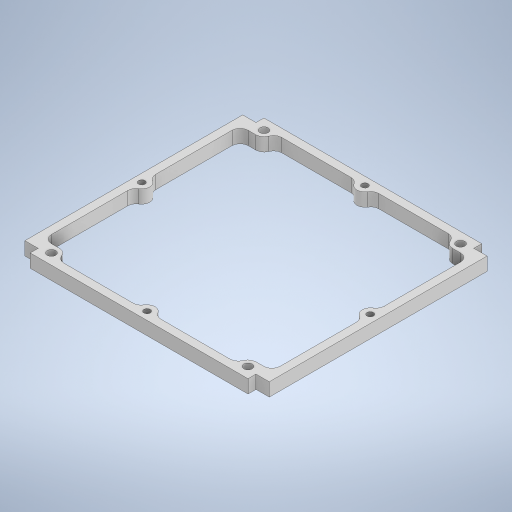
# Autodesk Inventor part: ElectronicsBayUpperMount
Saved by Autodesk Inventor 2023 (Build 270158000, 158)
## iProperties
Created: 2022-08-18
Part Number: ElectronicsBayUpperMount
Material: Generic
Document SubType Name: Modeling
Designer: Aditya Bansal
Density: 1 g/cm^3
Appearance: Default
Author: Aditya Bansal
Autodesk Inventor part; units mm, degrees
ref_plane "YZ Plane" through (0, 0, 0) normal (1, 0, 0) x (0, 1, 0)
ref_plane "XZ Plane" through (0, 0, 0) normal (0, 1, 0) x (-1, 0, 0)
ref_plane "XY Plane" through (0, 0, 0) normal (0, 0, 1) x (1, 0, 0)
sketch "Sketch1" plane through (0, 0, 0) normal (0, 1, 0) x (-1, 0, 0)
  line L0 (0, 0) -> (-92, 0)
  line L1 (-92, 0) -> (-92, -88)
  line L2 (-92, -88) -> (0, -88)
  line L3 (0, -88) -> (0, 0)
  line L4 (0, -88) -> (-5, -88)
  line L5 (-5, -88) -> (-5, -85)
  line L6 (-5, -85) -> (0, -85)
  line L7 (0, -85) -> (0, -88)
  line L8 (0, 0) -> (-5, 0)
  line L9 (-5, 0) -> (-5, -3)
  line L10 (-5, -3) -> (0, -3)
  line L11 (0, -3) -> (0, 0)
  line L12 (-92, 0) -> (-87, 0)
  line L13 (-87, 0) -> (-87, -3)
  line L14 (-87, -3) -> (-92, -3)
  line L15 (-92, -3) -> (-92, 0)
  line L16 (-92, -88) -> (-87, -88)
  line L17 (-87, -88) -> (-87, -85)
  line L18 (-87, -85) -> (-92, -85)
  line L19 (-92, -85) -> (-92, -88)
  circle A0 centre (-9, -84) radius 1.6 construction
  circle A1 centre (-83, -84) radius 1.6 construction
  circle A2 centre (-9, -4) radius 1.6 construction
  circle A3 centre (-83, -4) radius 1.6 construction
  circle A4 centre (-46, -85) radius 1.6 construction
  circle A5 centre (-3, -44) radius 1.6 construction
  circle A6 centre (-89, -44) radius 1.6 construction
  circle A7 centre (-46, -3) radius 1.6 construction
  circle A8 centre (-9, -84) radius 3
  circle A9 centre (-46, -85) radius 3
  circle A10 centre (-83, -84) radius 3
  circle A11 centre (-3, -44) radius 3
  circle A12 centre (-9, -4) radius 3
  circle A13 centre (-83, -4) radius 3
  circle A14 centre (-89, -44) radius 3
  circle A15 centre (-46, -3) radius 3
  line L20 (-11.8284, -3) -> (-43, -3)
  line L21 (-49, -3) -> (-80.1716, -3)
  line L22 (-83, -7) -> (-89, -7)
  line L23 (-89, -7) -> (-89, -41)
  line L24 (-83, -81) -> (-89, -81)
  line L25 (-89, -81) -> (-89, -47)
  line L26 (-80.1716, -85) -> (-49, -85)
  line L27 (-43, -85) -> (-11.8284, -85)
  line L28 (-9, -81) -> (-3, -81)
  line L29 (-9, -7) -> (-3, -7)
  line L30 (-3, -7) -> (-3, -41)
  line L31 (-3, -47) -> (-3, -81)
  point P0 (-92, -44)
  point P1 (-46, 0)
  dimension "d0" = 82
  dimension "d1" = 88
  dimension "d2" = 92
  dimension "d3" = 5
  dimension "d4" = 3.2
  dimension "d5" = 74
  dimension "d6" = 80
  dimension "d7" = 9
  dimension "d8" = 4
  dimension "d9" = 3.2
  dimension "d10" = 46
  dimension "d11" = 44
  dimension "d12" = 3
  dimension "d13" = 3
  dimension "d14" = 3
  dimension "d15" = 3
  dimension "d16" = 6
  dimension "d17" = 3
  dimension "d18" = 3
  dimension "d19" = 3
  dimension "d20" = 3
  constraints: 64 end point, 16 centre point, 16 point on circle, 13 equal radius, 12 parallel, 9 coincident, 8 horizontal, 8 perpendicular, 6 equal length, 6 point on line, 4 collinear, 3 horizontal alignment, 3 vertical alignment, 2 tangent
  measures "d0" distance between parallel lines of L14 L18
  measures "d1" distance between parallel lines of L2 L0
  measures "d2" distance between parallel lines of L3 L1
  measures "d3" distance of L18.start L18.end
  measures "d4" diameter of A0
  measures "d5" distance of A1.centre A0.centre
  measures "d6" distance of A2.centre A0.centre
  measures "d7" distance from line of A0.centre L3
  measures "d8" distance from line of L0 A2.centre
  measures "d9" diameter of A7
  measures "d10" distance from line of L1 A7.centre
  measures "d11" distance from line of L2 A6.centre
  measures "d12" distance from line of L0 A7.centre
  measures "d13" distance from line of L2 A4.centre
  measures "d14" distance from line of L1 A6.centre
  measures "d15" distance from line of L3 A5.centre
  measures "d16" diameter of A12
  measures "d17" distance between parallel lines of L0 L20
  measures "d18" distance between parallel lines of L3 L30
  measures "d19" distance between parallel lines of L27 L2
  measures "d20" distance between parallel lines of L1 L25
extrude "Extrusion1" add sketch "Sketch1" along normal blind 5 contours L9 L10 L3 A11 L30 L29 A12 L20 A15 L0 | A15 L21 A13 L22 L23 A14 L1 L14 L13 L0 | A15 | A11 | L3 L6 L5 L2 A9 L27 A8 L28 L31 A11 | A12 | A13 | A8 | A14 L25 L24 A10 L26 A9 L2 L17 L18 L1 | A14 | A9 | A10
fillet "Fillet1" radius 3 16 edges at (3, 2.5, -7) (11.8284, 2.5, -3) (43, 2.5, -3) (49, 2.5, -3) (80.1716, 2.5, -3) (89, 2.5, -7) (89, 2.5, -41) (89, 2.5, -47) (3, 2.5, -41) (3, 2.5, -47) (3, 2.5, -81) (11.8284, 2.5, -85) (43, 2.5, -85) (49, 2.5, -85) (89, 2.5, -81) (80.1716, 2.5, -85)
sketch "Sketch2" plane through (0, 5, 0) normal (0, 1, 0) x (1, 0, 0)
  arc A0 (87.5, 46.5981) -> (87.5, 41.4019) centre (89, 44) ccw projected
  arc A1 (43.4019, 83.5) -> (48.5981, 83.5) centre (46, 85) ccw projected
  arc A2 (4.5, 41.4019) -> (4.5, 46.5981) centre (3, 44) ccw projected
  arc A3 (48.5981, 4.5) -> (43.4019, 4.5) centre (46, 3) ccw projected
  point P0 (0, 0)
  point P1 (92, 44)
  point P2 (46, 0)
  constraints: 4 coincident
hole "Hole1" at (46, 5, -85) at (3, 5, -44) at (89, 5, -44) at (46, 5, -3) direction (0, -1, 0) diameter 2.459 end through all thread size "M3x0.5" class "6H" standard "ANSI Metric M Profile"
sketch "Sketch3" plane through (0, 5, 0) normal (0, 1, 0) x (1, 0, 0)
  arc A0 (9, 81) -> (11.8284, 83) centre (9, 84) ccw projected
  arc A1 (11.8284, 5) -> (9, 7) centre (9, 4) ccw projected
  arc A2 (80.1716, 83) -> (83, 81) centre (83, 84) ccw projected
  arc A3 (83, 7) -> (80.1716, 5) centre (83, 4) ccw projected
  point P0 (0, 0)
  point P1 (84, 6)
  constraints: 4 coincident, 1 other
hole "Hole2" at (9, 5, -84) at (9, 5, -4) at (83, 5, -4) at (83, 5, -84) direction (0, -1, 0) diameter 3.2 end through all clearance for "Flat Head Machine Screw" size "M3" standard "Ansi Metric M Profile"
equation "\"d7\" = -0.5 * d5 + 0.5 * d2"
equation "\"d8\" = -0.5 * d6 + 0.5 * d1"
equation "\"d10\" = 0.5 * d2"
equation "\"d11\" = 0.5 * d1"
equation "\"d13\" = d12"
equation "\"d15\" = d14"
equation "\"d17\" = d19"
equation "\"d18\" = d20"
body "Solid1"
